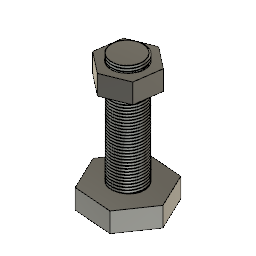
bolt-and-nut v1 (Autodesk Fusion 360 design; units mm, degrees)
Autodesk Fusion 360 part; units mm, degrees
sketch "Sketch1" plane through (0, 0, 0) normal (0, 0, 1) x (1, 0, 0) in component "bolt"
  line L0 (16.3462, 23.7936) -> (-12.4328, 26.053)
  line L1 (-12.4328, 26.053) -> (-28.779, 2.2594)
  line L2 (-28.779, 2.2594) -> (-16.3462, -23.7936)
  line L3 (-16.3462, -23.7936) -> (12.4328, -26.053)
  line L4 (12.4328, -26.053) -> (28.779, -2.2594)
  line L5 (28.779, -2.2594) -> (16.3462, 23.7936)
  circle A0 centre (0, 0) radius 12.5
  dimension "d1" = 25
  dimension "d2" = 50
  dimension "d3" = 25
  constraint coincident A0.centre origin
  measures "d1" distance of A0.centre L5
  measures "d2" distance of L2.end L4.end
  measures "d3" diameter of A0
extrude "Extrude1" add sketch "Sketch1" along normal blind 15 contours L0 L1 L2 L3 L4 L5 | A0 makes body 1 in component "bolt"
extrude "Extrude2" add sketch "Sketch1" along normal blind 100 contours A0 bodies 1 in component "bolt"
thread "Thread1" "ISO Metric profile 25.0 M25x2 6g" major diameter 24.822 minor diameter 22.5289 pitch 2 angle 60 modelled right hand crest width 0.2818 on face at (12.4379, 1.2446, 43.3333) crest through (12.411, 0, 14.5) on bodies 1 in component "bolt"
sketch "Sketch1 (2)" plane through (0, 0, 0) normal (0, 0, 1) x (1, 0, 0) in component "nut"
  line L0 (19.159, -7.7551) -> (16.2956, 12.7146)
  line L1 (16.2956, 12.7146) -> (-2.8634, 20.4697)
  line L2 (-2.8634, 20.4697) -> (-19.159, 7.7551)
  line L3 (-19.159, 7.7551) -> (-16.2956, -12.7146)
  line L4 (-16.2956, -12.7146) -> (2.8634, -20.4697)
  line L5 (2.8634, -20.4697) -> (19.159, -7.7551)
  circle A0 centre (0, 0) radius 12.5
  dimension "d11" = 25
  constraint coincident A0.centre origin
  measures "d11" diameter of A0
extrude "Extrude1'" add sketch "Sketch1 (2)" along normal blind 15 separate body makes body 2 in component "nut"
thread "Thread1'" "ISO Metric profile 25.0 M25x2 6H" major diameter 25.2565 minor diameter 23.0224 pitch 2 angle 60 modelled right hand crest width 0.5434 on face at (12.4379, -1.2446, 10) crest through (11.5112, 0, 0.5) on bodies 2 in component "nut"
component "bolt" placed x (1, 0, 0) y (0, 1, 0) z (0, 0, 1) at (0, 0, 0)
component "nut" placed x (1, 0, 0) y (0, -1, 0) z (0, 0, -1) at (-0.0007, 0.0498, 95)
